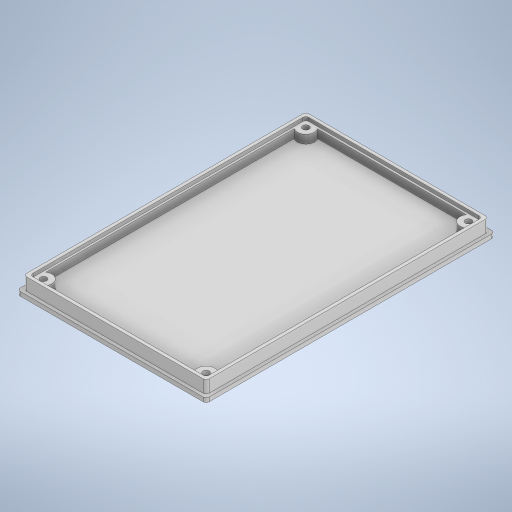
# Autodesk Inventor part: BoardMount
Saved by Autodesk Inventor 2023 (Build 270158000, 158)
## iProperties
Created: 2023-03-22
Part Number: BoardMount
Material: Generic
Document SubType Name: Modeling
Designer: User
Density: 1 g/cm^3
Appearance: Default
Author: User
Autodesk Inventor part; units mm, degrees
ref_plane "YZ Plane" through (0, 0, 0) normal (1, 0, 0) x (0, 1, 0)
ref_plane "XZ Plane" through (0, 0, 0) normal (0, 1, 0) x (-1, 0, 0)
ref_plane "XY Plane" through (0, 0, 0) normal (0, 0, 1) x (1, 0, 0)
sketch "Sketch1" plane through (0, 0, 0) normal (0, 1, 0) x (-1, 0, 0)
  line L0 (-45, 68.75) -> (45, 68.75)
  line L1 (45, 68.75) -> (45, -68.75)
  line L2 (45, -68.75) -> (-45, -68.75)
  line L3 (-45, -68.75) -> (-45, 68.75)
  line L4 (-45, 68.75) -> (45, -68.75) construction
  line L5 (45, 68.75) -> (-45, -68.75) construction
  point P0 (0, 0)
  dimension "d0" = 137.5
  dimension "d1" = 90
  constraints: 12 end point, 2 midpoint, 2 parallel, 1 horizontal, 1 perpendicular
  measures "d0" distance of L0.end L1.end
  measures "d1" distance of L1.end L2.end
extrude "Extrusion1" add sketch "Sketch1" along normal blind 8
sketch "Sketch2" plane through (0, 8, 0) normal (0, 1, 0) x (1, 0, 0)
  line L0 (42, -65.75) -> (-42, -65.75)
  line L1 (-42, -65.75) -> (-42, 65.75)
  line L2 (-42, 65.75) -> (42, 65.75)
  line L3 (42, 65.75) -> (42, -65.75)
  line L4 (42, -65.75) -> (-42, 65.75) construction
  line L5 (-42, -65.75) -> (42, 65.75) construction
  point P0 (0, 0)
  dimension "d4" = 131.5
  dimension "d5" = 84
  constraints: 12 end point, 2 midpoint, 2 parallel, 1 horizontal, 1 perpendicular
  measures "d4" distance of L0.end L1.end
  measures "d5" distance of L1.end L2.end
extrude "Extrusion2" cut sketch "Sketch2" against normal blind 1.6
sketch "Sketch3" plane through (0, 6.4, 0) normal (0, 1, 0) x (1, 0, 0)
  line L0 (41, -64.75) -> (-41, -64.75)
  line L1 (-41, -64.75) -> (-41, 64.75)
  line L2 (-41, 64.75) -> (41, 64.75)
  line L3 (41, 64.75) -> (41, -64.75)
  line L4 (41, -64.75) -> (-41, 64.75) construction
  line L5 (-41, -64.75) -> (41, 64.75) construction
  point P0 (0, 0)
  dimension "d8" = 129.5
  dimension "d9" = 82
  constraints: 12 end point, 2 midpoint, 2 parallel, 1 horizontal, 1 perpendicular
  measures "d8" distance of L0.end L1.end
  measures "d9" distance of L1.end L2.end
extrude "Extrusion3" cut sketch "Sketch3" against normal blind 4
sketch "Sketch4" plane through (0, 2.4, 0) normal (0, 1, 0) x (1, 0, 0)
  circle A0 centre (-38.75, -62.5) radius 4
  circle A1 centre (-38.75, 62.5) radius 4
  line L0 (41, -64.75) -> (-41, -64.75) projected
  circle A2 centre (38.75, -62.5) radius 4
  line L1 (41, 64.75) -> (41, -64.75) projected
  circle A3 centre (38.75, 62.5) radius 4
  line L2 (-41, -64.75) -> (-41, 64.75) projected
  point P0 (0, 0)
  point P1 (-41, -59.1928)
  point P2 (-35.4428, -64.75)
  point P3 (41, -59.1928)
  point P4 (35.4428, -64.75)
  dimension "d12" = 8
  dimension "d13" = 8
  dimension "d14" = 125
  dimension "d16" = 2.25
  dimension "d17" = 8
  dimension "d18" = 2.25
  dimension "d19" = 2.25
  dimension "d20" = 77.5
  dimension "d21" = 8
  dimension "d22" = 125
  dimension "d23" = 77.5
  dimension "d24" = 2.25
  constraints: 4 centre point
  measures "d12" diameter of A0
  measures "d13" diameter of A1
  measures "d14" distance of A1.centre A0.centre
  measures "d16" distance from line of L0 A0.centre
  measures "d17" diameter of A2
  measures "d18" distance from line of L1 A2.centre
  measures "d19" distance from line of L0 A2.centre
  measures "d20" distance of A2.centre A0.centre
  measures "d21" diameter of A3
  measures "d22" distance of A3.centre A2.centre
  measures "d23" distance of A3.centre A1.centre
  measures "d24" distance from line of L2 A1.centre
extrude "Extrusion4" add sketch "Sketch4" along normal blind 4 contours A0 L0 L2 | A3 | A2 L1 L0 | A1 picked at (-37.7393, -61.273) picked at (37.8547, -61.1739)
sketch "Sketch5" plane through (0, 6.4, 0) normal (0, 1, 0) x (1, 0, 0)
  arc A0 (-35.4428, -64.75) -> (-41, -59.1928) centre (-38.75, -62.5) ccw projected
  circle A1 centre (-38.75, -62.5) radius 1.5
  arc A2 (-41, 59.1928) -> (-35.4428, 64.75) centre (-38.75, 62.5) ccw projected
  circle A3 centre (-38.75, 62.5) radius 1.5
  arc A4 (35.4428, 64.75) -> (41, 59.1928) centre (38.75, 62.5) ccw projected
  circle A5 centre (38.75, 62.5) radius 1.5
  arc A6 (41, -59.1928) -> (35.4428, -64.75) centre (38.75, -62.5) ccw projected
  circle A7 centre (38.75, -62.5) radius 1.5
  point P0 (0, 0)
  dimension "d27" = 3
  dimension "d28" = 3
  dimension "d29" = 3
  dimension "d30" = 3
  constraints: 4 centre point, 4 coincident
  measures "d27" diameter of A1
  measures "d28" diameter of A3
  measures "d29" diameter of A5
  measures "d30" diameter of A7
extrude "Extrusion5" cut sketch "Sketch5" against normal blind 4
fillet "Fillet1" radius 1.5 4 edges at (-42, 7.2, 65.75) (-42, 7.2, -65.75) (42, 7.2, 65.75) (42, 7.2, -65.75)
sketch "Sketch6" plane through (0, 8, 0) normal (0, 1, 0) x (1, 0, 0)
  line L0 (43.5, -67.25) -> (-43.5, -67.25)
  line L1 (-43.5, -67.25) -> (-43.5, 67.25)
  line L2 (-43.5, 67.25) -> (43.5, 67.25)
  line L3 (43.5, 67.25) -> (43.5, -67.25)
  line L4 (43.5, -67.25) -> (-43.5, 67.25) construction
  line L5 (-43.5, -67.25) -> (43.5, 67.25) construction
  line L6 (45.5, -69.25) -> (-45.5, -69.25)
  line L7 (-45.5, -69.25) -> (-45.5, 69.25)
  line L8 (-45.5, 69.25) -> (45.5, 69.25)
  line L9 (45.5, 69.25) -> (45.5, -69.25)
  line L10 (45.5, -69.25) -> (-45.5, 69.25) construction
  line L11 (-45.5, -69.25) -> (45.5, 69.25) construction
  point P0 (0, 0)
  dimension "d35" = 134.5
  dimension "d36" = 87
  dimension "d37" = 138.5
  dimension "d38" = 91
  constraints: 24 end point, 4 midpoint, 4 parallel, 2 horizontal, 2 perpendicular
  measures "d35" distance of L0.end L1.end
  measures "d36" distance of L1.end L2.end
  measures "d37" distance of L6.end L7.end
  measures "d38" distance of L7.end L8.end
extrude "Extrusion6" cut sketch "Sketch6" against normal blind 6
fillet "Fillet3" radius 1.5 8 edges at (43.5, 5, 67.25) (45, 1, 68.75) (43.5, 5, -67.25) (45, 1, -68.75) (-43.5, 5, -67.25) (-45, 1, -68.75) (-43.5, 5, 67.25) (-45, 1, 68.75)
body "Solid1"
